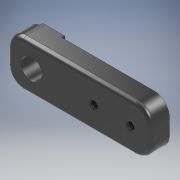
# Autodesk Inventor part: Frame_Z_Endstop_Mount_LM3048
Saved by Autodesk Inventor 2020.3 (Build 243373000, 373)
## iProperties
Created: 2020-06-09
Part Number: Frame_Z_Endstop_Mount_LM3048
Material: ABS Plastic
Document SubType Name: Modeling
Designer: rah75
Density: 1.06 g/cm^3
Appearance: Satin - Black
Author: rah75
Autodesk Inventor part; units mm, degrees
ref_plane "YZ Plane" through (0, 0, 0) normal (1, 0, 0) x (0, 1, 0)
ref_plane "XZ Plane" through (0, 0, 0) normal (0, 1, 0) x (-1, 0, 0)
ref_plane "XY Plane" through (0, 0, 0) normal (0, 0, 1) x (1, 0, 0)
sketch "Sketch1" plane through (0, 0, 0) normal (0, 0, 1) x (1, 0, 0)
  line L0 (-18.5, -6) -> (18.5, -6)
  line L1 (18.5, -6) -> (18.5, 6)
  line L2 (18.5, 6) -> (-18.5, 6)
  line L3 (-18.5, 6) -> (-18.5, -6)
  line L4 (-18.5, -6) -> (18.5, 6) construction
  line L5 (18.5, -6) -> (-18.5, 6) construction
  point P0 (0, 0)
  dimension "d0" = 37
  dimension "d1" = 12
  constraints: 12 end point, 2 midpoint, 2 parallel, 1 horizontal, 1 perpendicular
  measures "d0" distance of L1.end L2.end
  measures "d1" distance of L0.end L1.end
extrude "Extrusion1" add sketch "Sketch1" along normal mid plane 5
sketch "Sketch2" plane through (-18.5, 6, 2.5) normal (0, 1, 0) x (1, 0, 0)
  line L0 (3.2, 5.874) -> (9.2, 5.874)
  line L1 (9.2, 5.874) -> (9.2, 4.874)
  line L2 (9.2, 4.874) -> (3.2, 4.874)
  line L3 (3.2, 4.874) -> (3.2, 5.874)
  line L4 (3.2, 5.874) -> (9.2, 4.874) construction
  line L5 (9.2, 5.874) -> (3.2, 4.874) construction
  line L6 (37, 5) -> (37, 0) projected
  line L7 (9.074, 5.748) -> (3.326, 5.748)
  line L8 (3.326, 5.748) -> (3.326, 5)
  line L9 (3.326, 5) -> (9.074, 5)
  line L10 (9.074, 5) -> (9.074, 5.748)
  line L11 (0, 5) -> (37, 5) projected
  point P0 (18.5, 2.5)
  point P1 (6.2, 5.374)
  dimension "d4" = 27.8
  dimension "d5" = 1
  dimension "d6" = 6
  dimension "d7" = 0.126
  constraints: 20 end point, 4 parallel, 2 midpoint, 2 perpendicular, 1 collinear, 1 horizontal, 3 other
  measures "d4" distance between parallel lines of L6 L1
  measures "d5" distance of L0.end L1.end
  measures "d6" distance of L0.start L0.end
  measures "d7" distance between parallel lines of L0 L7
extrude "Extrusion2" add sketch "Sketch2" against normal up to surface (12 mm away) contours L8 L7 L10 L9
sketch "Sketch3" plane through (0, 0, 2.5) normal (0, 0, 1) x (1, 0, 0)
  line L0 (-18.5, -6) -> (18.5, -6) projected
  line L1 (-9.426, -6) -> (-15.174, -6) projected
  line L2 (-15.174, 6) -> (-15.174, -6) projected
  line L3 (-9.426, 6) -> (-15.174, 6) projected
  line L4 (-9.426, 6) -> (-9.426, -6) projected
  point P0 (0, 0)
  point P1 (-12.3, 0)
  point P2 (-12.3, 6)
  point P3 (-9.426, 0)
  constraints: 2 midpoint, 1 horizontal alignment, 1 vertical alignment
hole "Hole1" at (-12.3, 0, 2.5) direction (0, 0, -1) diameter 5.5 depth 14.2 clearance for "Socket Head Cap Screw" size "M5" standard "Ansi Metric M Profile"
fillet "Fillet1" radius 4 4 edges at (-18.5, 6, 0) (-18.5, -6, 0) (18.5, -6, 0) (18.5, 6, 0)
fillet "Fillet2" radius 1 8 edges at (-17.3284, 4.8284, 2.5) (-18.5, 0, 2.5) (-17.3284, -4.8284, 2.5) (0, -6, 2.5) (17.3284, -4.8284, 2.5) (18.5, 0, 2.5) (17.3284, 4.8284, 2.5) (0, 6, 2.5)
sketch "Sketch4" plane through (0, 0, -2.5) normal (0, 0, -1) x (-1, 0, 0)
  line L0 (-18.5, 2) -> (-18.5, -2) projected
  point P0 (0, 0)
  point P1 (-13.4, 0)
  point P2 (-3.9, 0)
  dimension "d19" = 5.1
  dimension "d20" = 14.6
  constraints: 2 horizontal alignment
  measures "d19" distance from line of L0 point (-13.4, 0)
  measures "d20" distance from line of L0 point (-3.9, 0)
hole "Hole2" at (13.4, 0, -2.5) at (3.9, 0, -2.5) direction (0, 0, 1) diameter 2.013 depth 7.6 thread size "M2.5x0.45" class "6H" standard "ANSI Metric M Profile"
body "Solid1"
